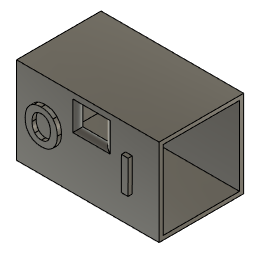
temperature & humidity (Autodesk Fusion 360 design; units mm, degrees)
Autodesk Fusion 360 part; units mm, degrees
sketch "Sketch1" plane through (0, 0, 0) normal (0, 0, 1) x (1, 0, 0)
  line L0 (16.7, 9.2) -> (-16.7, 9.2)
  line L1 (-16.7, 9.2) -> (-16.7, -9.2)
  line L2 (-16.7, -9.2) -> (16.7, -9.2)
  line L3 (16.7, -9.2) -> (16.7, 9.2)
  line L4 (16.7, 9.2) -> (-16.7, -9.2) construction
  line L5 (-16.7, 9.2) -> (16.7, -9.2) construction
  line L6 (-17.7, -10.2) -> (17.7, -10.2)
  line L7 (17.7, -10.2) -> (17.7, 10.2)
  line L8 (17.7, 10.2) -> (-17.7, 10.2)
  line L9 (-17.7, 10.2) -> (-17.7, -10.2)
  dimension "d1" = 33.4
  dimension "d2" = 18.4
  dimension "d3" = 1
  constraint horizontal L0
  constraint perpendicular L0 L1
  constraint parallel L0 L2
  constraint parallel L1 L3
  constraint coincident L4 origin
  constraint coincident L5 origin
  measures "d1" distance of L1.end L2.end
  measures "d2" distance of L0.end L1.end
extrude "Extrude1" add sketch "Sketch1" against normal blind 1 contours L0 L1 L2 L3 | L6 L7 L8 L9 makes body 1
extrude "Extrude2" add sketch "Sketch1" along normal blind 18 bodies 1
sketch "Sketch2" plane through (0, 0, 18) normal (0, 0, 1) x (-1, 0, 0)
  line L0 (-16.7, -9.2) -> (-16.7, 9.2)
  line L1 (-16.7, 9.2) -> (16.7, 9.2)
  line L2 (16.7, 9.2) -> (16.7, -9.2)
  line L3 (16.7, -9.2) -> (-16.7, -9.2)
  line L4 (17.7, -10.2) -> (17.7, 10.2)
  line L5 (17.7, 10.2) -> (-17.7, 10.2)
  line L6 (-17.7, 10.2) -> (-17.7, -10.2)
  line L7 (-17.7, -10.2) -> (17.7, -10.2)
extrude "Extrude3" add sketch "Sketch2" along normal blind 1 contours L0 L1 L2 L3 | L4 L5 L6 L7 bodies 1
sketch "Sketch3" plane through (17.7, 0, 0) normal (1, 0, 0) x (0, 1, 0)
  line L0 (-10.2, 19) -> (-10.2, -1)
  line L1 (-10.2, -1) -> (10.2, -1)
  line L2 (10.2, -1) -> (10.2, 19)
  line L3 (10.2, 19) -> (-10.2, 19)
  line L4 (9.2, 0) -> (-9.2, 0)
  line L5 (-9.2, 0) -> (-9.2, 18)
  line L6 (-9.2, 18) -> (9.2, 18)
  line L7 (9.2, 18) -> (9.2, 0)
  constraint horizontal L4
  constraint vertical L5
  constraint horizontal L6
  constraint vertical L7
extrude "Extrude4" cut sketch "Sketch3" against normal blind 2 contours L4 L5 L6 L7 bodies 1
extrude "Extrude5" cut 2 faces at (17.0333, -3.0667, 18) (5.5667, -3.0667, 18) along direction (0, 0, 1) blind 1 on bodies 1 bodies 1
sketch "Sketch4" plane through (0, 0, 19) normal (0, 0, 1) x (-1, 0, 0)
  line L0 (-17.7, 9.2) -> (16.7, 9.2)
  line L1 (16.7, 9.2) -> (16.7, -9.2)
  line L2 (16.7, -9.2) -> (-17.7, -9.2)
  line L3 (-17.7, -9.2) -> (-17.7, -10.2)
  line L4 (-17.7, -10.2) -> (17.7, -10.2)
  line L5 (17.7, -10.2) -> (17.7, 10.2)
  line L6 (17.7, 10.2) -> (-17.7, 10.2)
  line L7 (-17.7, 10.2) -> (-17.7, 9.2)
  line L8 (17.7, -10.2) -> (-17.7, -10.2)
  line L9 (-17.7, -10.2) -> (-17.7, 10.2)
  line L10 (-17.7, 10.2) -> (17.7, 10.2)
  line L11 (17.7, 10.2) -> (17.7, -10.2)
  constraint horizontal L8
  constraint vertical L9
  constraint horizontal L10
  constraint vertical L11
  constraint coincident L6.end L7.start
  constraint coincident L4.end L5.start
extrude "Extrude6" add sketch "Sketch4" along normal blind 1 bodies 1
sketch "Sketch5" plane through (-17.7, 0, 0) normal (-1, 0, 0) x (0, -1, 0)
  line L0 (-10.2, 20) -> (-10.2, -1)
  line L1 (-10.2, -1) -> (10.2, -1)
  line L2 (10.2, -1) -> (10.2, 20)
  line L3 (10.2, 20) -> (-10.2, 20)
  line L4 (10.2, 0.0678) -> (10.2, 3.4678)
  line L5 (-10.2, -0.0375) -> (-7.2, -0.0375)
  line L6 (10.2, 0.0678) -> (6.2, 0.0678)
  line L7 (10.2, 3.4678) -> (-10.2, 3.4678) construction
  line L8 (-7.2, -0.0375) -> (-7.2, 3.4678) construction
  line L9 (6.2, 0.0678) -> (6.2, 3.4678) construction
  line L10 (-7.2, 3.4678) -> (6.1981, 3.4678) construction
  line L11 (6.1981, 3.4678) -> (6.1981, 18.4678) construction
  line L12 (6.1981, 18.4678) -> (-7.2, 18.4678) construction
  line L13 (-7.2, 18.4678) -> (-7.2, 3.4678) construction
  line L14 (-7.2, 18.4678) -> (6.1981, 18.4678) construction
  line L15 (6.1981, 18.4678) -> (6.1981, 3.4678) construction
  line L16 (6.1981, 3.4678) -> (-7.2, 3.4678) construction
  line L17 (-7.2, 3.4678) -> (-7.2, 18.4678) construction
  line L18 (-7.2, 18.4678) -> (6.1981, 18.4678)
  line L19 (6.1981, 18.4678) -> (6.1981, 3.4678)
  line L20 (6.1981, 3.4678) -> (-7.2, 3.4678)
  line L21 (-7.2, 3.4678) -> (-7.2, 18.4678)
  dimension "d16" = 3.4
  dimension "d17" = 3
  dimension "d18" = 4
  dimension "d19" = 15
  constraint coincident L2 L4.start
  constraint parallel L2 L4
  constraint coincident L0 L5.start
  constraint perpendicular L0 L5
  constraint perpendicular L2 L6
  constraint coincident L0 L7.end
  constraint perpendicular L0 L7
  constraint coincident L7 L8.end
  constraint perpendicular L7 L8
  constraint coincident L7 L9.end
  constraint perpendicular L7 L9
  constraint horizontal L10
  constraint vertical L11
  constraint horizontal L12
  constraint vertical L13
  constraint horizontal L14
  constraint vertical L15
  constraint horizontal L16
  constraint vertical L17
  constraint horizontal L18
  constraint vertical L19
  constraint horizontal L20
  constraint vertical L21
  measures "d16" distance of L4.start L4.end
  measures "d17" distance of L5.start L5.end
  measures "d18" distance of L4.start L6.end
  measures "d19" distance of L8.end L12.end
extrude "Extrude7" cut sketch "Sketch5" against normal blind 1.5 contours L18 L19 L20 L21 bodies 1
extrude "Extrude8" add 1 faces at (-17.0333, -1.7321, 18.4678) along direction (0, 0, -1) blind 0.2 on bodies 1 bodies 1
sketch "Sketch6" plane through (0, -10.2, 0) normal (0, -1, 0) x (1, 0, 0)
  line L0 (-17.7, 20) -> (-17.7, -1)
  line L1 (-17.7, -1) -> (17.7, -1)
  line L2 (17.7, -1) -> (17.7, 20)
  line L3 (17.7, 20) -> (-17.7, 20)
  line L4 (-16.7, 0) -> (0.4, 0) construction
  line L5 (0.4, 0) -> (0.4, 19) construction
  line L6 (1, 0) -> (1, 15) construction
  line L7 (2.4, 17) -> (-1.6, 17)
  line L8 (-1.6, 17) -> (-1.6, 13)
  line L9 (-1.6, 13) -> (2.4, 13)
  line L10 (2.4, 13) -> (2.4, 17)
  line L11 (2.4, 17) -> (-1.6, 13) construction
  line L12 (-1.6, 17) -> (2.4, 13) construction
  line L13 (-1.6, 17) -> (2.4, 17)
  line L14 (2.4, 17) -> (2.4, 18.8)
  line L15 (2.4, 18.8) -> (-1.6, 18.8)
  line L16 (-1.6, 18.8) -> (-1.6, 17)
  point P0 (0.4, 15)
  dimension "d24" = 17.1
  dimension "d25" = 4
  dimension "d26" = 4
  constraint horizontal L4
  constraint perpendicular L4 L5
  constraint parallel L5 L6
  constraint horizontal L7
  constraint perpendicular L7 L8
  constraint parallel L7 L9
  constraint parallel L8 L10
  constraint coincident L11 P0
  constraint coincident L12 P0
  constraint coincident L5 P0
  constraint horizontal L13
  constraint vertical L14
  constraint horizontal L15
  constraint vertical L16
  measures "d24" distance of L4.start L4.end
  measures "d25" distance of L8.end L9.end
  measures "d26" distance of L7.end L8.end
extrude "Extrude9" cut sketch "Sketch6" against normal blind 2 contours L7 L8 L9 L10 L13 bodies 1
fillet "Fillet1" radius 0.1 4 edges at (-1.6, -10.2, 15) (0.4, -10.2, 17) (2.4, -10.2, 15) (0.4, -10.2, 13) on bodies 1
sketch "Sketch7" plane through (-16.7, 0, 0) normal (1, 0, 0) x (0, 1, 0)
  line L0 (-6.1981, 3.4678) -> (-6.1981, 18.2678)
  line L1 (-6.1981, 18.2678) -> (7.2, 18.2678)
  line L2 (7.2, 18.2678) -> (7.2, 3.4678)
  line L3 (7.2, 3.4678) -> (-6.1981, 3.4678)
  line L4 (-9.2, 0) -> (9.2, 0)
  line L5 (9.2, 0) -> (9.2, 19)
  line L6 (9.2, 19) -> (-9.2, 19)
  line L7 (-9.2, 19) -> (-9.2, 0)
  line L8 (-6.1981, 3.4678) -> (-9.2, 3.4678)
  line L9 (-9.2, 3.4678) -> (-9.2, 4.4678)
  line L10 (-9.2, 4.4678) -> (-6.1981, 4.4678)
  line L11 (-6.1981, 4.4678) -> (-6.1981, 3.4678)
  line L12 (7.2, 3.4678) -> (9.2, 3.4678)
  line L13 (9.2, 3.4678) -> (9.2, 4.4678)
  line L14 (9.2, 4.4678) -> (7.2, 4.4678)
  line L15 (7.2, 4.4678) -> (7.2, 3.4678)
  dimension "d31" = 1
  constraint horizontal L8
  constraint vertical L9
  constraint horizontal L10
  constraint vertical L11
  constraint coincident L7 L9.end
  constraint coincident L0.start L3.end
  constraint horizontal L12
  constraint vertical L13
  constraint horizontal L14
  constraint vertical L15
  constraint coincident L5 L13.end
  constraint coincident L2.end L3.start
  measures "d31" distance of L0.start L10.end
extrude "Extrude10" add sketch "Sketch7" along normal blind 3 contours L0 L7 L8 L9 L10 L11 | L2 L5 L12 L13 L14 L15 bodies 1
extrude "Extrude11" cut 1 faces at (17.7, -9.8667, 12.6667) along direction (-1, 0, 0) blind 1 on bodies 1 bodies 1
sketch "Sketch8" plane through (16.7, 0, 0) normal (1, 0, 0) x (0, 1, 0)
  line L0 (9.2, 19) -> (9.2, 0)
  line L1 (9.2, 0) -> (-9.2, 0)
  line L2 (-9.2, 0) -> (-9.2, 19)
  line L3 (-9.2, 19) -> (9.2, 19)
  line L4 (10.2, -1) -> (10.2, 20)
  line L5 (10.2, 20) -> (-10.2, 20)
  line L6 (-10.2, 20) -> (-10.2, -1)
  line L7 (-10.2, -1) -> (10.2, -1)
ref_plane "WorkPlane1" through (23.7, 0, 9.5) normal (1, 0, 0) x (0, 1, 0)
sketch "Sketch9" plane through (23.7, 0, 9.5) normal (1, 0, 0) x (0, 1, 0)
  line L0 (-10.2, 10.5) -> (10.2, 10.5)
  line L1 (10.2, 10.5) -> (10.2, -10.5)
  line L2 (10.2, -10.5) -> (-10.2, -10.5)
  line L3 (-10.2, -10.5) -> (-10.2, 10.5)
  line L4 (-6.2, 8.77) -> (7.2, 8.77)
  line L5 (7.2, 8.77) -> (7.2, -6.0325)
  line L6 (7.2, -6.0325) -> (-6.2, -6.0325)
  line L7 (-6.2, -6.0325) -> (-6.2, 8.77)
  constraint horizontal L0
  constraint vertical L1
  constraint horizontal L2
  constraint vertical L3
  constraint horizontal L4
  constraint vertical L5
  constraint horizontal L6
  constraint vertical L7
extrude "Extrude12" add sketch "Sketch9" along normal blind 1 separate body makes body 2
sketch "Sketch10" plane through (23.7, 0, 0) normal (-1, 0, 0) x (0, -1, 0)
  line L0 (6.2, 3.4675) -> (-7.2, 3.4675)
  line L1 (-7.2, 3.4675) -> (-7.2, 18.27)
  line L2 (-7.2, 18.27) -> (6.2, 18.27)
  line L3 (6.2, 18.27) -> (6.2, 3.4675)
  line L4 (-10.2, -1) -> (10.2, -1)
  line L5 (10.2, -1) -> (10.2, 20)
  line L6 (10.2, 20) -> (-10.2, 20)
  line L7 (-10.2, 20) -> (-10.2, -1)
  line L8 (9.2, 19) -> (-9.2, 19)
  line L9 (-9.2, 19) -> (-9.2, 0)
  line L10 (-9.2, 0) -> (9.2, 0)
  line L11 (9.2, 0) -> (9.2, 19)
  line L12 (-8.2, 19) -> (-8.2, 1)
  line L13 (-8.2, 1) -> (8.2, 1)
  line L14 (8.2, 1) -> (8.2, 19)
  line L15 (-8.2, 18.27) -> (8.2, 18.27)
  dimension "d39" = -1
  constraint horizontal L8
  constraint vertical L9
  constraint horizontal L10
  constraint vertical L11
  constraint coincident L12 L15.start
  constraint coincident L14 L15.end
  constraint perpendicular L14 L15
extrude "Extrude13" add sketch "Sketch10" along normal blind 2 contours L2 L8 L12 L14 L15 | L8 L9 L10 L11 L12 L13 L14 bodies 2
sketch "Sketch11" plane through (21.7, 0, 0) normal (-1, 0, 0) x (0, -1, 0)
  line L0 (8.2, 1) -> (-8.2, 1)
  line L1 (-8.2, 1) -> (-8.2, 18.27)
  line L2 (-8.2, 18.27) -> (8.2, 18.27)
  line L3 (8.2, 18.27) -> (8.2, 1)
  line L4 (9.2, 0) -> (9.2, 19)
  line L5 (9.2, 19) -> (-9.2, 19)
  line L6 (-9.2, 19) -> (-9.2, 0)
  line L7 (-9.2, 0) -> (9.2, 0)
  line L8 (-9.2, 3.4677) -> (-8.2, 3.4677)
  line L9 (-8.2, 3.4677) -> (-8.2, 1.8677)
  line L10 (-8.2, 1.8677) -> (-9.2, 1.8677)
  line L11 (-9.2, 1.8677) -> (-9.2, 3.4677)
  line L12 (9.2, 3.4678) -> (8.2, 3.4678)
  line L13 (8.2, 3.4678) -> (8.2, 1.8678)
  line L14 (8.2, 1.8678) -> (9.2, 1.8678)
  line L15 (9.2, 1.8678) -> (9.2, 3.4678)
  dimension "d42" = 1.6
  dimension "d43" = 1.6
  constraint horizontal L8
  constraint vertical L9
  constraint horizontal L10
  constraint vertical L11
  constraint coincident L1 L9.end
  constraint coincident L6 L8.start
  constraint horizontal L12
  constraint vertical L13
  constraint horizontal L14
  constraint vertical L15
  constraint coincident L3 L13.end
  constraint coincident L4 L12.start
  measures "d42" distance of L8.start L10.end
  measures "d43" distance of L12.start L14.end
extrude "Extrude14" cut sketch "Sketch11" against normal blind 2 contours L3 L4 L12 L13 L14 L15 | L1 L6 L8 L9 L10 L11 bodies 2
extrude "Extrude15" cut 1 faces at (1.0667, -9.8, 17) along direction (0, 0, 1) blind 1.6 on bodies 1 bodies 1
sketch "Sketch12" plane through (0, -10.2, 0) normal (0, -1, 0) x (1, 0, 0)
  line L0 (16.7, -1) -> (16.7, 20)
  line L1 (16.7, 20) -> (-17.7, 20)
  line L2 (-17.7, 20) -> (-17.7, -1)
  line L3 (-17.7, -1) -> (16.7, -1)
  line L4 (-1.7, 17.1) -> (2.5, 17.1)
  line L5 (2.5, 17.1) -> (2.5, 12.9)
  line L6 (2.5, 12.9) -> (-1.7, 12.9)
  line L7 (-1.7, 12.9) -> (-1.7, 17.1)
extrude "Extrude16" cut sketch "Sketch6" against normal blind 0.4 contours L7 L13 L14 L15 L16 bodies 1
extrude "Extrude17" add 1 faces at (1.0667, -10.0667, 18.8) along direction (0, 0, -1) blind 0.2 on bodies 1 bodies 1
extrude "Extrude18" cut 1 faces at (-1.6, -9.5, 16.2) along direction (-1, 0, 0) blind 0.1 on bodies 1 bodies 1
extrude "Extrude19" cut 2 faces at (2.4, -10.1333, 17.5667) (2.4, -9.5, 16.2) along direction (1, 0, 0) blind 0.1 on bodies 1 bodies 1
delete_face "DeleteFace1" 1 faces at (2.4936, -10.1998, 14.3063) on bodies 1
sketch "Sketch13" plane through (0, -10.2, 0) normal (0, -1, 0) x (1, 0, 0)
  line L0 (-1.7, 17.1) -> (-1.7, 18.6)
  line L1 (-1.7, 18.6) -> (2.5, 18.6)
  line L2 (2.5, 18.6) -> (2.5, 17.1)
  line L3 (2.5, 17.1) -> (-1.7, 17.1)
  line L4 (-17.7, 20) -> (-17.7, -1)
  line L5 (-17.7, -1) -> (16.7, -1)
  line L6 (16.7, -1) -> (16.7, 20)
  line L7 (16.7, 20) -> (-17.7, 20)
  line L8 (-1.7, 17.1) -> (2.5, 17.1)
  line L9 (2.5, 17.1) -> (2.5, 13)
  line L10 (2.5, 13) -> (-1.7, 13)
  line L11 (-1.7, 13) -> (-1.7, 17.1)
  constraint horizontal L8
  constraint vertical L9
  constraint horizontal L10
  constraint vertical L11
  constraint coincident L0.start L3.end
extrude "Extrude20" cut sketch "Sketch13" against normal blind 1 contours L3 L8 L9 L10 L11 bodies 1
extrude "Extrude21" cut 2 faces at (2.5, -9.5, 16.2) (2.5, -10.1333, 14.3333) along direction (1, 0, 0) blind 1 on bodies 1 bodies 1
extrude "Extrude22" cut 1 faces at (-1.7, -9.5333, 16.2333) along direction (-1, 0, 0) blind 1 on bodies 1 bodies 1
fillet "Fillet2" radius 1.5 3 edges at (-2.7, -10.2, 15.8) (0.4, -10.2, 13) (3.5, -10.2, 15.8) on bodies 1
sketch "Sketch14" plane through (0, -10.2, 0) normal (0, -1, 0) x (1, 0, 0)
  line L0 (-17.7, 20) -> (-17.7, -1)
  line L1 (-17.7, -1) -> (16.7, -1)
  line L2 (16.7, -1) -> (16.7, 20)
  line L3 (16.7, 20) -> (-17.7, 20)
  line L4 (-4.1142, 18.6) -> (4.9142, 18.6)
  line L5 (4.9142, 18.6) -> (4.9142, 11.5858)
  line L6 (4.9142, 11.5858) -> (-4.1142, 11.5858)
  line L7 (-4.1142, 11.5858) -> (-4.1142, 18.6)
  line L8 (-15.1056, 10.2361) -> (-10.5631, 10.2361) construction
  line L9 (-10.5631, 10.2361) -> (-10.5631, 16.0765) construction
  line L10 (-10.5631, 16.0765) -> (-15.1056, 16.0765) construction
  line L11 (-15.1056, 16.0765) -> (-15.1056, 10.2361) construction
  line L12 (-15.1056, 10.2361) -> (-10.5631, 10.2361) construction
  line L13 (-10.5631, 10.2361) -> (-10.5631, 16.0765) construction
  line L14 (-10.5631, 16.0765) -> (-15.1056, 16.0765) construction
  line L15 (-15.1056, 16.0765) -> (-15.1056, 10.2361) construction
  line L16 (8.5956, 7.6887) -> (12.6757, 7.6739) construction
  line L17 (12.6757, 7.6739) -> (12.6982, 13.88) construction
  line L18 (12.6982, 13.88) -> (8.618, 13.8948) construction
  line L19 (8.618, 13.8948) -> (8.5956, 7.6887) construction
  text T0 "O" font "Arial" height 8 bold align left top in box 4.5426 x 5.8404 at (-15.1056, 10.2361) x (1, 0) y (0, 1) spacing 1 kerned
  text T1 "I\n" font "Arial" height 8 bold align left top in box 4.0802 x 6.2061 at (8.5956, 7.6887) x (0.999993, -0.003614) y (0.003614, 0.999993) spacing 1 kerned
extrude "Extrude23" add sketch "Sketch14" along normal blind 1 text T0 bodies 1
extrude "Extrude24" add sketch "Sketch14" along normal blind 1 text T1 bodies 1
hidden bodies 2
